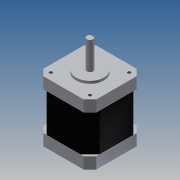
# Autodesk Inventor part: stepper
Saved by Autodesk Inventor 2013 (Build 170138000, 138)
## iProperties
Created: 2017-03-28
Part Number: stepper
Material: Generic
Document SubType Name: Modeling
Designer: employee
Density: 1 g/cm^3
Author: employee
Autodesk Inventor part; units mm, degrees
ref_plane "YZ Plane" through (0, 0, 0) normal (1, 0, 0) x (0, 1, 0)
ref_plane "XZ Plane" through (0, 0, 0) normal (0, 1, 0) x (-1, 0, 0)
ref_plane "XY Plane" through (0, 0, 0) normal (0, 0, 1) x (1, 0, 0)
sketch "Sketch1" plane through (0, 0, 0) normal (0, 0, 1) x (1, 0, 0)
  line L0 (-21, 21) -> (21, 21)
  line L1 (21, 21) -> (21, -21)
  line L2 (21, -21) -> (-21, -21)
  line L3 (-21, -21) -> (-21, 21)
  point P0 (0, 0)
  point P1 (0, 0)
  dimension "d0" = 42
  constraints: 8 end point, 1 coincident, 1 horizontal, 9 other
  measures "d0" distance of L0.start L0.end
extrude "Extrusion1" add sketch "Sketch1" along normal mid plane 48
sketch "Sketch2" plane through (0, 0, 24) normal (0, 0, 1) x (1, 0, 0)
  circle A0 centre (0, 0) radius 11
  dimension "d3" = 22
  constraints: 1 centre point, 1 coincident
  measures "d3" diameter of A0
extrude "Extrusion2" add sketch "Sketch2" along normal blind 2
sketch "Sketch3" plane through (0, 0, 26) normal (0, 0, 1) x (1, 0, 0)
  circle A0 centre (0, 0) radius 11 projected
  circle A1 centre (0, 0) radius 2.5
  dimension "d7" = 5
  constraints: 1 centre point, 1 coincident
  measures "d7" diameter of A1
extrude "Extrusion3" add sketch "Sketch3" along normal blind 22 contours A1
sketch "Sketch4" plane through (0, 0, 48) normal (0, 0, 1) x (1, 0, 0)
  circle A0 centre (0, 0) radius 2.5 projected
  line L0 (-1.5, 2) -> (1.5, 2)
  dimension "d11" = 2
  constraints: 2 end point, 2 point on circle, 1 horizontal
  measures "d11" distance from line of L0 A0.centre
extrude "Extrusion4" cut sketch "Sketch4" against normal blind 15 contours L0 A0 picked at (-0.3466, 2.0912)
sketch "Sketch5" plane through (0, 0, 24) normal (0, 0, 1) x (1, 0, 0)
  circle A0 centre (0, 0) radius 11 projected
  line L0 (-15.5, 15.5) -> (15.5, 15.5)
  line L1 (15.5, 15.5) -> (15.5, -15.5)
  line L2 (15.5, -15.5) -> (-15.5, -15.5)
  line L3 (-15.5, -15.5) -> (-15.5, 15.5)
  dimension "d14" = 31
  constraints: 8 end point, 1 coincident, 1 horizontal, 9 other
  measures "d14" distance of L0.start L0.end
hole "Hole1" at (-15.5, 15.5, 24) at (15.5, 15.5, 24) at (15.5, -15.5, 24) at (-15.5, -15.5, 24) direction (0, 0, -1) diameter 2.459 end through all thread size "M3x0.5" class "6H" standard "ANSI Metric M Profile"
chamfer "Chamfer1" distance 5 angle 45 4 edges at (21, 21, 0) (-21, 21, 0) (21, -21, 0) (-21, -21, 0)
sketch "Sketch6" plane through (0, 0, 0) normal (0, 0, 1) x (1, 0, 0)
  line L0 (-21, 16) -> (-16, 21) projected
  line L1 (-16, 21) -> (16, 21) projected
  line L2 (16, 21) -> (21, 16) projected
  line L3 (21, 16) -> (21, -16) projected
  line L4 (21, -16) -> (16, -21) projected
  line L5 (16, -21) -> (-16, -21) projected
  line L6 (-16, -21) -> (-21, -16) projected
  line L7 (-21, -16) -> (-21, 16) projected
  circle A0 centre (15.5, -15.5) radius 1.2295 projected
  circle A1 centre (-15.5, 15.5) radius 1.2295 projected
  circle A2 centre (15.5, 15.5) radius 1.2295 projected
  circle A3 centre (-15.5, -15.5) radius 1.2295 projected
  line L8 (-21, 13.1716) -> (-13.1716, 21)
  point P0 (0, 0)
  dimension "d25" = 2
  constraints: 2 end point, 2 point on line, 1 perpendicular
  measures "d25" distance between parallel lines of L0 L8
extrude "Extrusion5" cut sketch "Sketch6" along normal mid plane 30 contours L0 L1 L8 L7
pattern_circular "Circular Pattern1" count 4 over 360 about axis through (0, 0, 26) along (0, 0, 1) of "Extrusion5"
sketch "Sketch7" plane through (-16, -21, 24) normal (0, -1, 0) x (1, 0, 0)
  line L0 (-5, -39) -> (-5, -9) projected
  line L1 (-5, -39) -> (2.8284, -39) projected
  line L2 (2.8284, -9) -> (2.8284, -39) projected
  line L3 (2.8284, -9) -> (-5, -9) projected
  line L4 (29.1716, -39) -> (29.1716, -9) projected
  line L5 (29.1716, -39) -> (37, -39) projected
  line L6 (37, -9) -> (37, -39) projected
  line L7 (37, -9) -> (29.1716, -9) projected
  line L8 (-5, -9) -> (37, -9)
  line L9 (37, -9) -> (37, -39)
  line L10 (37, -39) -> (-5, -39)
  line L11 (-5, -39) -> (-5, -9)
  point P0 (16, -24)
  constraints: 8 end point, 2 parallel, 1 horizontal, 1 perpendicular
extrude "Extrusion6" cut sketch "Sketch7" against normal blind 0.1
pattern_circular "Circular Pattern2" count 4 over 360 about axis through (0, 0, 26) along (0, 0, 1) of "Extrusion6"
body "Solid1"
